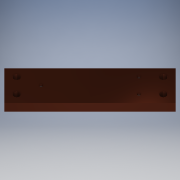
# Autodesk Inventor part: mount-base
Saved by Autodesk Inventor 2017 SP1 (Build 210196100, 196)
## iProperties
Created: 2017-02-03
Part Number: mount-base
Material: Copper
Document SubType Name: Modeling
Designer: Alex
Density: 8.94 g/cm^3
Appearance: Copper - Polished
Author: Alex
Autodesk Inventor part; units mm, degrees
ref_plane "YZ Plane" through (0, 0, 0) normal (1, 0, 0) x (0, 1, 0)
ref_plane "XZ Plane" through (0, 0, 0) normal (0, 1, 0) x (-1, 0, 0)
ref_plane "XY Plane" through (0, 0, 0) normal (0, 0, 1) x (1, 0, 0)
sketch "Sketch1" plane through (0, 0, 0) normal (0, 1, 0) x (-1, 0, 0)
  line L0 (-10, 25) -> (-10, 0)
  line L1 (10, 0) -> (10, 25)
  line L2 (10, 0) -> (-10, 0) construction
  line L3 (10, 30) -> (-10, 30) construction
  line L4 (10, 25) -> (-10, 25) construction
  line L5 (0, 25) -> (0, 0) construction
  line L6 (10, 20) -> (-10, 20) construction
  line L7 (10, 20) -> (0, 20) construction
  line L8 (0, 20) -> (-10, 20) construction
  line L9 (0, 20) -> (5, 20) construction
  line L10 (0, 20) -> (-5, 20) construction
  line L11 (10, 35) -> (10, 25)
  line L12 (-10, 35) -> (-10, 25)
  line L13 (10, 35) -> (-10, 35)
  line L14 (5, 35) -> (5, 30)
  line L15 (-5, 35) -> (-5, 30)
  line L16 (-10, -25) -> (-10, 0)
  line L17 (10, 0) -> (10, -25)
  line L18 (10, -30) -> (-10, -30) construction
  line L19 (10, -25) -> (-10, -25) construction
  line L20 (0, -25) -> (0, 0) construction
  line L21 (10, -20) -> (-10, -20) construction
  line L22 (10, -20) -> (0, -20) construction
  line L23 (0, -20) -> (-10, -20) construction
  line L24 (0, -20) -> (5, -20) construction
  line L25 (0, -20) -> (-5, -20) construction
  line L26 (10, -35) -> (10, -25)
  line L27 (-10, -35) -> (-10, -25)
  line L28 (10, -35) -> (-10, -35)
  line L29 (5, -35) -> (5, -30)
  line L30 (-5, -35) -> (-5, -30)
  dimension "d84" = 5
  dimension "d127" = 20
  constraints: 62 end point, 16 symmetric about line, 12 point on line, 8 midpoint, 5 perpendicular, 2 collinear, 1 horizontal, 1 parallel, 1 vertical
  measures "d84" distance between parallel lines of L6 L4
  measures "d127" distance between parallel lines of L0 L1
extrude "Extrusion1" add sketch "Sketch1" along normal blind 5
hole "Hole12" at (-5, 0, 30) at (5, 0, 30) at (-5, 0, -30) at (5, 0, -30) direction (0, 1, 0) diameter 3.4 end through all clearance for "Socket Head Cap Screw ISO 4762" size "M3" standard "ISO"
hole "Hole13" at (0, 0, 20) at (-5, 0, -20) at (5, 0, -20) direction (0, 1, 0) diameter 1.567 end through all thread size "M2x0.4" class "6H" standard "ISO Metric profile"
body "Solid1"
